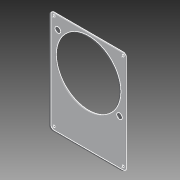
# Autodesk Inventor part: raspi-holder-top
Saved by Autodesk Inventor 2014 (Build 180170000, 170)
## iProperties
Created: 2017-08-16
Part Number: raspi-holder-top
Material: 一般
Document SubType Name: Modeling
Designer: hide
Density: 1 g/cm^3
Appearance: 既定
Author: hide
Autodesk Inventor part; units mm, degrees
ref_plane "YZ Plane" through (0, 0, 0) normal (1, 0, 0) x (0, 1, 0)
ref_plane "XZ Plane" through (0, 0, 0) normal (0, 1, 0) x (-1, 0, 0)
ref_plane "XY Plane" through (0, 0, 0) normal (0, 0, 1) x (1, 0, 0)
sketch "スケッチ1" plane through (0, 0, 0) normal (0, 1, 0) x (-1, 0, 0)
  line L0 (0, 0) -> (68, 0)
  line L1 (68, 0) -> (68, 92)
  line L2 (68, 92) -> (0, 92)
  line L3 (0, 92) -> (0, 0)
  circle A0 centre (3, 89) radius 0.9
  circle A1 centre (3, 3) radius 0.9
  circle A2 centre (65, 3) radius 0.9
  circle A3 centre (65, 89) radius 0.9
  circle A4 centre (34, 60) radius 29
  circle A5 centre (61.6925, 79.7262) radius 0.9
  circle A6 centre (6.2481, 40.3574) radius 0.9
  line L4 (6.2481, 40.3574) -> (71.1751, 86.4594)
  dimension "d0" = 92
  dimension "d1" = 68
  dimension "d2" = 3
  dimension "d3" = 3
  dimension "d4" = 1.8
  dimension "d5" = 1.8
  dimension "d6" = 3
  dimension "d7" = 3
  dimension "d8" = 1.8
  dimension "d9" = 3
  dimension "d10" = 3
  dimension "d11" = 3
  dimension "d12" = 3
  dimension "d13" = 1.8
  dimension "d17" = 58
  dimension "d18" = 32
  dimension "d19" = 34
  dimension "d20" = 1.8
  dimension "d21" = 1.8
  dimension "d24" = 34
  dimension "d25" = 34
  constraints: 10 end point, 7 centre point, 2 parallel, 1 horizontal, 1 perpendicular, 1 point on line
  measures "d0" distance of L2.end L0.start
  measures "d1" distance of L1.end L2.end
  measures "d2" distance from line of A3.centre L1
  measures "d3" distance from line of L2 A3.centre
  measures "d4" diameter of A3
  measures "d5" diameter of A0
  measures "d6" distance from line of A0.centre L2
  measures "d7" distance from line of A0.centre L3
  measures "d8" diameter of A2
  measures "d9" distance from line of A2.centre L1
  measures "d10" distance from line of A2.centre L0
  measures "d11" distance from line of A1.centre L0
  measures "d12" distance from line of A1.centre L3
  measures "d13" diameter of A1
  measures "d17" diameter of A4
  measures "d18" distance from line of A4.centre L2
  measures "d19" distance from line of A4.centre L3
  measures "d20" diameter of A5
  measures "d21" diameter of A6
  measures "d24" distance of A4.centre A5.centre
  measures "d25" distance of A4.centre L4.start
extrude "押し出し1" add sketch "スケッチ1" along normal blind 1.3
fillet "フィレット1" radius 3 4 edges at (0, 0.65, 92) (0, 0.65, 0) (-68, 0.65, 0) (-68, 0.65, 92)
sketch "スケッチ2" plane through (0, 1.3, 0) normal (0, 1, 0) x (1, 0, 0)
  circle A0 centre (-6.2481, -40.3574) radius 0.9 projected
  circle A1 centre (-61.6925, -79.7262) radius 0.9 projected
  circle A2 centre (-6.2481, -40.3574) radius 2.5
  circle A3 centre (-61.6925, -79.7262) radius 2.5
  point P0 (0, 0)
  dimension "d26" = 5
  dimension "d27" = 5
  constraints: 2 centre point, 2 coincident
  measures "d26" diameter of A2
  measures "d27" diameter of A3
extrude "押し出し2" add sketch "スケッチ2" along normal blind 4
sketch "スケッチ3" plane through (0, 1.3, 0) normal (0, 1, 0) x (1, 0, 0)
  line L0 (-45.9767, -23.6507) -> (-43.3974, -22.1186)
  line L1 (-43.3974, -22.1186) -> (-39.3119, -28.9967)
  line L2 (-39.3119, -28.9967) -> (-41.8911, -30.5288)
  line L3 (-41.8911, -30.5288) -> (-45.9767, -23.6507)
  line L4 (-63, -33.7624) -> (-60.4207, -32.2303)
  line L5 (-60.4207, -32.2303) -> (-56.3352, -39.1084)
  line L6 (-56.3352, -39.1084) -> (-58.9145, -40.6405)
  line L7 (-58.9145, -40.6405) -> (-63, -33.7624)
  point P0 (0, 0)
  dimension "d31" = 8
  dimension "d32" = 8
  dimension "d33" = 3
  dimension "d34" = 3
  dimension "d35" = 0
  dimension "d46" = 22.8
  constraints: 16 end point, 4 parallel, 2 perpendicular
  measures "d31" distance of L2.end L0.start
  measures "d32" distance of L4.end L5.end
  measures "d33" distance between parallel lines of L3 L1
  measures "d34" distance between parallel lines of L5 L7
  measures "d35" distance between parallel lines of L6 L2
  measures "d46" distance between parallel lines of L7 L1
extrude "押し出し3" [suppressed]
sketch "スケッチ6" plane through (0, 1.3, 0) normal (0, 1, 0) x (1, 0, 0)
  line L0 (-43.3974, -22.1186) -> (-39.3119, -28.9967) projected
  line L1 (-58.9145, -40.6405) -> (-63, -33.7624) projected
  line L2 (-58.9145, -40.6405) -> (-63, -33.7624)
  line L3 (-63, -33.7624) -> (-64.7195, -34.7838)
  line L4 (-64.7195, -34.7838) -> (-60.634, -41.6619)
  line L5 (-60.634, -41.6619) -> (-58.9145, -40.6405)
  line L6 (-39.3119, -28.9967) -> (-43.3974, -22.1186)
  line L7 (-43.3974, -22.1186) -> (-41.6779, -21.0972)
  line L8 (-41.6779, -21.0972) -> (-37.5923, -27.9753)
  line L9 (-37.5923, -27.9753) -> (-39.3119, -28.9967)
  line L10 (-64.0424, -28.8936) -> (-47.7828, -19.2356)
  line L11 (-47.7828, -19.2356) -> (-47.0244, -20.5124)
  line L12 (-47.0244, -20.5124) -> (-63.284, -30.1705)
  line L13 (-63.284, -30.1705) -> (-64.0424, -28.8936)
  point P0 (0, 0)
  dimension "d47" = 2
  dimension "d48" = 2
  constraints: 24 end point, 8 equal length, 4 perpendicular
  measures "d47" distance between parallel lines of L2 L4
  measures "d48" distance between parallel lines of L6 L8
extrude "押し出し6" [suppressed]
sketch "スケッチ7" plane through (0, 4.8, 0) normal (0, 1, 0) x (1, 0, 0)
  line L0 (-58.9145, -40.6405) -> (-63, -33.7624) projected
  line L1 (-64.7195, -34.7838) -> (-60.634, -41.6619) projected
  line L2 (-43.3974, -22.1186) -> (-39.3119, -28.9967) projected
  line L3 (-39.3119, -28.9967) -> (-37.5923, -27.9753) projected
  line L4 (-37.5923, -27.9753) -> (-41.6779, -21.0972) projected
  line L5 (-41.6779, -21.0972) -> (-43.3974, -22.1186) projected
  line L6 (-64.7195, -34.7838) -> (-60.634, -41.6619)
  line L7 (-60.634, -41.6619) -> (-58.0547, -40.1298)
  line L8 (-58.0547, -40.1298) -> (-62.1402, -33.2517)
  line L9 (-62.1402, -33.2517) -> (-64.7195, -34.7838)
  line L10 (-41.6779, -21.0972) -> (-37.5461, -28.0532)
  line L11 (-37.5461, -28.0532) -> (-40.1254, -29.5852)
  line L12 (-40.1254, -29.5852) -> (-44.2572, -22.6293)
  line L13 (-44.2572, -22.6293) -> (-41.6779, -21.0972)
  point P0 (0, 0)
  dimension "d51" = 3
  dimension "d52" = 3
  constraints: 16 end point, 5 parallel, 2 perpendicular, 1 point on line
  measures "d51" distance between parallel lines of L10 L12
  measures "d52" distance between parallel lines of L1 L8
extrude "押し出し7" [suppressed]
equation "\"d3\" = d2"
equation "\"d5\" = d4"
equation "\"d6\" = d3"
equation "\"d7\" = d3"
equation "\"d8\" = d4"
equation "\"d9\" = d2"
equation "\"d10\" = d2"
equation "\"d11\" = d2"
equation "\"d12\" = d2"
equation "\"d13\" = d4"
equation "\"d19\" = 0.5 * d1"
equation "\"d21\" = d20"
equation "\"d25\" = d24"
equation "\"d27\" = d26"
equation "\"d32\" = d31"
equation "\"d34\" = d33"
equation "\"d48\" = d47"
equation "\"d52\" = d51"
